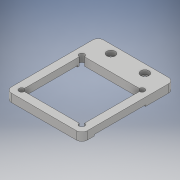
# Autodesk Inventor part: Metal_mount_horizontal_coverslip22x22_v2
Saved by Autodesk Inventor 2017 (Build 210142000, 142)
## iProperties
Created: 2019-10-14
Part Number: Metal_mount_horizontal_coverslip22x22_v2
Material: Generic
Document SubType Name: Modeling
Designer: nvladim
Density: 1 g/cm^3
Appearance: Default
Author: nvladim
Autodesk Inventor part; units mm, degrees
ref_plane "YZ Plane" through (0, 0, 0) normal (1, 0, 0) x (0, 1, 0)
ref_plane "XZ Plane" through (0, 0, 0) normal (0, 1, 0) x (-1, 0, 0)
ref_plane "XY Plane" through (0, 0, 0) normal (0, 0, 1) x (1, 0, 0)
sketch "Sketch1" plane through (0, 0, 0) normal (0, 1, 0) x (-1, 0, 0)
  line L0 (-11.1, -11.1) -> (-10.1, -11.1)
  line L1 (11.1, -11.1) -> (11.1, -10.1)
  line L2 (11.1, 11.1) -> (10.1, 11.1)
  line L3 (-11.1, 11.1) -> (-11.1, 10.1)
  line L4 (-11.1, -11.1) -> (11.1, 11.1) construction
  line L5 (11.1, -11.1) -> (-11.1, 11.1) construction
  line L6 (-14, -14) -> (14, -14)
  line L7 (14, -14) -> (14, 14)
  line L8 (14, 14) -> (-14, 14)
  line L9 (-14, 14) -> (-14, -14)
  line L10 (-14, -14) -> (14, 14) construction
  line L11 (14, -14) -> (-14, 14) construction
  line L12 (14, 14) -> (20, 14)
  line L13 (20, 14) -> (20, -14)
  line L14 (20, -14) -> (14, -14)
  line L15 (14, -14) -> (14, 14)
  line L16 (3.6361, 0) -> (-5.9421, 0)
  circle A0 centre (11.1, 11.1) radius 1
  line L17 (0, 4.2823) -> (0, -4.7782)
  circle A1 centre (11.1, -11.1) radius 1
  circle A2 centre (-11.1, 11.1) radius 1
  circle A3 centre (-11.1, -11.1) radius 1
  line L18 (11.1, 10.1) -> (11.1, 11.1)
  line L19 (10.1, 11.1) -> (-10.1, 11.1)
  line L20 (11.1, -10.1) -> (11.1, 10.1)
  line L21 (10.1, -11.1) -> (11.1, -11.1)
  line L22 (-11.1, 10.1) -> (-11.1, -10.1)
  line L23 (-10.1, 11.1) -> (-11.1, 11.1)
  line L24 (-10.1, -11.1) -> (10.1, -11.1)
  line L25 (-11.1, -10.1) -> (-11.1, -11.1)
  point P0 (0, 0)
  point P1 (17, 6.25)
  point P2 (17, -6.25)
  dimension "d0" = 22.2
  dimension "d1" = 22.2
  dimension "d2" = 28
  dimension "d3" = 28
  dimension "d4" = 6
  dimension "d5" = 12.5
  dimension "d6" = 2
  dimension "d9" = 22.2
  dimension "d12" = 22.2
  dimension "d17" = 3
  constraints: 52 end point, 22 parallel, 12 perpendicular, 8 point on circle, 7 horizontal, 4 centre point, 4 midpoint, 1 coincident, 1 symmetric about line, 1 vertical, 6 other
  measures "d0" distance of L3.start L2.start
  measures "d1" distance of L2.start L1.start
  measures "d2" distance of L8.end L7.end
  measures "d3" distance of L7.end L6.end
  measures "d4" distance of L13.end L14.end
  measures "d5" diameter of point (17, 6.25) L16
  measures "d6" diameter of A0
  measures "d9" distance of A0.centre A1.centre
  measures "d12" distance of A0.centre A2.centre
  measures "d17" distance from line of L7 point (17, 6.25)
extrude "Extrusion1" add sketch "Sketch1" along normal blind 3
hole "Hole1" at (-17, 0, 6.25) at (-17, 0, -6.25) direction (0, 1, 0) diameter 3.1 end through all countersink diameter 6 countersink angle 90
fillet "Fillet1" radius 2 2 edges at (14, 1.5, -14) (14, 1.5, 14)
fillet "Fillet2" radius 2 2 edges at (-20, 1.5, -14) (-20, 1.5, 14)
sketch "Sketch2" plane through (0, 0, 0) normal (0, -1, 0) x (1, 0, 0)
  line L0 (12, -14) -> (-18, -14) projected
  line L1 (-9.5, 14) -> (9.5, 14)
  line L2 (9.5, 14) -> (9.5, -14)
  line L3 (9.5, -14) -> (-9.5, -14)
  line L4 (-9.5, -14) -> (-9.5, 14)
  line L5 (-9.5, 14) -> (9.5, -14) construction
  line L6 (9.5, 14) -> (-9.5, -14) construction
  point P0 (0, 0)
  dimension "d27" = 19
  constraints: 12 end point, 2 midpoint, 2 parallel, 1 horizontal, 1 perpendicular, 1 point on line
  measures "d27" distance of L2.end L3.end
extrude "Extrusion2" cut sketch "Sketch2" against normal blind 0.5
body "Solid1"
